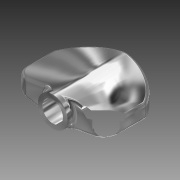
# Autodesk Inventor part: button
Saved by Autodesk Inventor 2014 (Build 180170000, 170)
## iProperties
Shininess: 86.0
Length Units: 11272
Angle Units: 11279
Time Units: 11290
Mass Units: 11286
Length Display Precision: 3
Angle Display Precision: 2
Compacted: True
Created: 2001-07-10
Part Number: button
Document SubType Name: Modeling
Designer: Autodesk, Inc.
Mass: 10.3635 g
Surface Area: 11.0347 cm^2
Volume: 1.28261 cm^3
Density: 8.08 g/cm^3
Material: Stainless Steel
Appearance: Chrome - Polished
Density: 0.0
Volumn: 0.0
Area: 0.0
PropertySet Name: Model Information
Control State: 0
Master: False
Checked Out: False
Author: Autodesk, Inc.
Autodesk Inventor part; units mm, degrees
ref_plane "YZ Plane" through (0, 0, 0) normal (1, 0, 0) x (0, 1, 0)
ref_plane "XZ Plane" through (0, 0, 0) normal (0, 1, 0) x (-1, 0, 0)
ref_plane "XY Plane" through (0, 0, 0) normal (0, 0, 1) x (1, 0, 0)
ref_plane "Work Plane1" through (0, 0, 0) normal (0, 0, 1) x (1, 0, 0)
sketch "Sketch2" plane through (0, 0, 0) normal (0, 0, 1) x (1, 0, 0)
  circle A0 centre (-0.360296, 0) radius 2.38125
  circle A1 centre (-0.360296, 0) radius 3.444875
  line L0 (-0.360296, 0) -> (-0.360296, 7.9375) construction
  line L1 (-0.360296, 0) -> (-19.05, 0) construction
  line L2 (-11.1125, 1.5875) -> (-0.963227, 3.391701)
  line L3 (10.391909, 1.5875) -> (0.242635, 3.391701)
  line L4 (-11.1125, -1.5875) -> (-0.963227, -3.391701)
  line L5 (10.391909, -1.5875) -> (0.242635, -3.391701)
  circle A2 centre (-0.360296, 0) radius 2.38125
  circle A3 centre (-0.360296, 0) radius 3.444875
  arc A4 (0.242635, -3.391701) -> (0.242635, 3.391701) centre (-0.360296, 0) ccw
  line L6 (-11.1125, 1.5875) -> (-11.1125, -1.5875)
  line L7 (10.391909, 1.5875) -> (10.391909, -1.5875)
  arc A5 (-0.963227, 3.391701) -> (-0.963227, -3.391701) centre (-0.360296, 0) ccw
  constraints: 16 end point, 7 coincident, 6 point on circle, 6 symmetric about line, 4 centre point, 2 perpendicular, 2 point on line, 1 concentric, 1 parallel, 1 vertical, 7 other
extrude "Extrusion1" add sketch "Sketch2" along normal mid plane 3.175 contours A1
extrude "Extrusion2" add sketch "Sketch2" against normal blind 15.875
fillet "Fillet1" radius 3.175 2 edges at (10.3919, 0, 0) (-11.1125, 0, 0)
fillet "Fillet2" radius 0.762 3 edges at (2.2802, -2.2125, 0) (2.2802, 2.2125, 0) (-3.8052, 0, 0)
sketch "Sketch3" plane through (0, 0, 0) normal (0, 1, 0) x (-1, 0, 0)
  line L0 (-10.391909, 0) -> (-10.391909, -15.875)
  line L1 (11.1125, 0) -> (11.1125, -15.875)
  line L2 (-3.084579, 1.5875) -> (3.805171, 1.5875)
  arc A0 (-10.1603, -9.781928) -> (10.885715, -9.720151) centre (0.344022, -3.385388) ccw
  line L3 (-13.200856, -8.956267) -> (-13.200856, -17.299941)
  line L4 (-13.200856, -17.299941) -> (12.993124, -17.299941)
  line L5 (12.993124, -17.299941) -> (12.993124, -8.902464)
  arc A1 (-10.391909, -8.956267) -> (-10.1603, -9.781928) centre (-8.804409, -8.956267) ccw
  line L6 (-8.804409, -8.956267) -> (-13.200856, -8.956267)
  line L7 (0.344022, -3.385388) -> (0.344022, -4.550959)
  arc A2 (10.885715, -9.720151) -> (11.1125, -8.902464) centre (9.525, -8.902464) ccw
  line L8 (9.525, -8.902464) -> (12.993124, -8.902464)
  dimension "d12" = 3.175
  dimension "d13" = 3.175
  constraints: 12 end point, 6 point on circle, 4 tangent, 3 centre point, 2 perpendicular, 2 point on line, 1 parallel, 1 other
  measures "d12" diameter of A1
  measures "d13" diameter of A2
extrude "Extrusion3" cut sketch "Sketch3" against normal mid plane 15.875
fillet "Fillet3" radius 0.762 22 edges at (10.3919, 1.5875, -6.0656) (10.3919, -1.5875, -6.0656) (9.462, 1.7528, -0.9299) (4.9185, 2.5605, 0) (1.4147, 3.1833, 0.2475) (9.462, -1.7528, -0.9299) (4.9185, -2.5605, 0) (1.4147, -3.1833, 0.2475) (-6.6675, 2.3777, -13.9338) (-11.1125, 1.5875, -6.0387) (-10.1826, 1.7528, -0.9299) (-5.6391, 2.5605, 0) (-2.1353, 3.1833, 0.2475) (-0.3603, 3.4449, -15.684) (5.9345, 2.3799, -13.9607) (5.9345, -2.3799, -13.9607) (-0.3589, -3.4449, -15.684) (-6.6675, -2.3777, -13.9338) (-2.1353, -3.1833, 0.2475) (-5.6391, -2.5605, 0) (-10.1826, -1.7528, -0.9299) (-11.1125, -1.5875, -6.0387)
body "Solid1"
